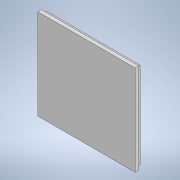
# Autodesk Inventor part: lid
Saved by Autodesk Inventor 2022 (Build 260153070, 153G)
## iProperties
Created: 2021-07-10
Part Number: lid
Material: 常规
Document SubType Name: Modeling
Designer: peter
Density: 1 g/cm^3
Appearance: 默认
Author: peter
Autodesk Inventor part; units mm, degrees
ref_plane "YZ Plane" through (0, 0, 0) normal (1, 0, 0) x (0, 1, 0)
ref_plane "XZ Plane" through (0, 0, 0) normal (0, 1, 0) x (-1, 0, 0)
ref_plane "XY Plane" through (0, 0, 0) normal (0, 0, 1) x (1, 0, 0)
sketch "草图1" plane through (0, 0, 0) normal (0, 0, 1) x (1, 0, 0)
  line L0 (-173.6, 0) -> (-39.6, 0)
  line L1 (-39.6, 0) -> (-39.6, 124)
  line L2 (-39.6, 124) -> (-173.6, 124)
  line L3 (-173.6, 124) -> (-173.6, 0)
  point P0 (0, 0)
  dimension "d0" = 124
  dimension "d1" = 134
  constraints: 8 end point, 2 parallel, 1 horizontal, 1 perpendicular
  measures "d0" distance between parallel lines of L0 L2
  measures "d1" distance between parallel lines of L3 L1
extrude "拉伸1" add sketch "草图1" along normal blind 5
sketch "草图3" plane through (0, 0, 5) normal (0, 0, 1) x (1, 0, 0)
  line L0 (-176.6, 127) -> (-36.6, 127)
  line L1 (-36.6, 127) -> (-36.6, -3)
  line L2 (-36.6, -3) -> (-176.6, -3)
  line L3 (-176.6, -3) -> (-176.6, 127)
  line L4 (-39.6, 124) -> (-173.6, 124) projected
  line L5 (-39.6, 0) -> (-39.6, 124) projected
  line L6 (-173.6, 0) -> (-39.6, 0) projected
  line L7 (-173.6, 124) -> (-173.6, 0) projected
  point P0 (0, 0)
  dimension "d4" = 3
  dimension "d5" = 3
  dimension "d6" = 3
  dimension "d7" = 3
  constraints: 8 end point, 2 parallel, 1 horizontal, 1 perpendicular
  measures "d4" distance between parallel lines of L4 L0
  measures "d5" distance between parallel lines of L5 L1
  measures "d6" distance between parallel lines of L6 L2
  measures "d7" distance between parallel lines of L3 L7
extrude "拉伸2" add sketch "草图3" along normal blind 5 contours L0 L1 L2 L3 | L5 L6 L7 L4
